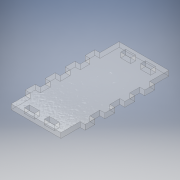
# Autodesk Inventor part: case_side
Saved by Autodesk Inventor 2019 (Build 230136000, 136)
## iProperties
Created: 2019-02-02
Part Number: case_side
Material: Acrylic, Clear
Document SubType Name: Modeling
Designer: suchanek
Density: 1.19 g/cm^3
Appearance: Transparent - Clear
Author: suchanek
Autodesk Inventor part; units mm, degrees
ref_plane "YZ Plane" through (0, 0, 0) normal (1, 0, 0) x (0, 1, 0)
ref_plane "XZ Plane" through (0, 0, 0) normal (0, 1, 0) x (-1, 0, 0)
ref_plane "XY Plane" through (0, 0, 0) normal (0, 0, 1) x (1, 0, 0)
sketch "Sketch1" plane through (0, 0, 0) normal (0, 1, 0) x (-1, 0, 0)
  line L0 (30, 65) -> (-30, 65)
  line L1 (-30, 65) -> (-30, -65)
  line L2 (-30, -65) -> (30, -65)
  line L3 (30, -65) -> (30, 65)
  line L4 (30, 65) -> (-30, -65) construction
  line L5 (-30, 65) -> (30, -65) construction
  line L6 (-18, 61) -> (-6, 61)
  line L7 (-6, 61) -> (-6, 55)
  line L8 (-6, 55) -> (-18, 55)
  line L9 (-18, 55) -> (-18, 61)
  line L10 (-30, 6) -> (-36, 6)
  line L11 (-36, 6) -> (-36, 18)
  line L12 (-36, 18) -> (-30, 18)
  line L13 (-30, 18) -> (-30, 6)
  line L14 (-30, 30) -> (-36, 30)
  line L15 (-36, 30) -> (-36, 42)
  line L16 (-36, 42) -> (-30, 42)
  line L17 (-30, 42) -> (-30, 30)
  line L18 (0, 0) -> (0, 6.5854)
  line L19 (0, 6.5854) -> (0, 0)
  line L20 (0, 0) -> (-5.5856, 0)
  line L21 (18, 61) -> (6, 61)
  line L22 (6, 61) -> (6, 55)
  line L23 (6, 55) -> (18, 55)
  line L24 (18, 55) -> (18, 61)
  line L25 (30, 6) -> (36, 6)
  line L26 (36, 6) -> (36, 18)
  line L27 (36, 18) -> (30, 18)
  line L28 (30, 18) -> (30, 6)
  line L29 (30, 30) -> (36, 30)
  line L30 (36, 30) -> (36, 42)
  line L31 (36, 42) -> (30, 42)
  line L32 (30, 42) -> (30, 30)
  line L33 (-18, -61) -> (-6, -61)
  line L34 (-6, -61) -> (-6, -55)
  line L35 (-6, -55) -> (-18, -55)
  line L36 (-18, -55) -> (-18, -61)
  line L37 (-30, -6) -> (-36, -6)
  line L38 (-36, -6) -> (-36, -18)
  line L39 (-36, -18) -> (-30, -18)
  line L40 (-30, -18) -> (-30, -6)
  line L41 (-30, -30) -> (-36, -30)
  line L42 (-36, -30) -> (-36, -42)
  line L43 (-36, -42) -> (-30, -42)
  line L44 (-30, -42) -> (-30, -30)
  line L45 (6, -55) -> (18, -55)
  line L46 (18, -61) -> (6, -61)
  line L47 (6, -61) -> (6, -55)
  line L48 (18, -55) -> (18, -61)
  line L49 (30, -18) -> (30, -6)
  line L50 (36, -42) -> (30, -42)
  line L51 (36, -30) -> (36, -42)
  line L52 (30, -6) -> (36, -6)
  line L53 (36, -6) -> (36, -18)
  line L54 (30, -42) -> (30, -30)
  line L55 (36, -18) -> (30, -18)
  line L56 (30, -30) -> (36, -30)
  dimension "d0" = 60
  dimension "d1" = 130
  dimension "d2" = 6
  dimension "d3" = 12
  dimension "d4" = 12
  dimension "d5" = 12
  dimension "d6" = 6
  dimension "d9" = 4
  dimension "d10" = 6
  dimension "d13" = 12
  dimension "d14" = 12
  constraints: 114 end point, 36 symmetric about line, 9 equal length, 6 point on line, 5 horizontal, 4 perpendicular, 2 midpoint, 1 vertical
  measures "d0" distance of L0.start L0.end
  measures "d1" distance of L2.end L0.start
  measures "d2" distance between parallel lines of L10 L20
  measures "d3" distance of L10.end L11.end
  measures "d4" distance between parallel lines of L14 L12
  measures "d5" distance of L14.end L15.end
  measures "d6" distance of L10.start L10.end
  measures "d9" distance between parallel lines of L0 L6
  measures "d10" distance of L8.end L6.start
  measures "d13" distance between parallel lines of L7 L22
  measures "d14" distance of L6.start L6.end
extrude "Extrusion1" add sketch "Sketch1" along normal blind 6
body "Solid1"
